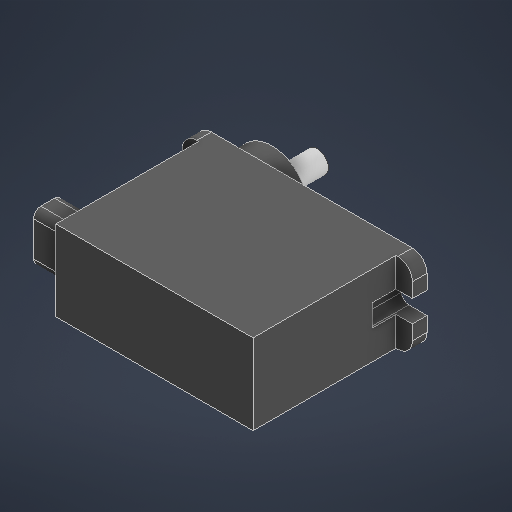
# Autodesk Inventor part: P_Servo_SIMPROP_27x12
Saved by Autodesk Inventor 2026 (Build 300175000, 175)
## iProperties
Created: 2025-08-29
Part Number: P_Servo_SIMPROP_27x12
Material: Generisch
Document SubType Name: Modeling
Designer: FAL
Density: 1 g/cm^3
Appearance: Vorgabe
Author: FAL
Autodesk Inventor part; units mm, degrees
ref_plane "YZ Plane" through (0, 0, 0) normal (1, 0, 0) x (0, 1, 0)
ref_plane "XZ Plane" through (0, 0, 0) normal (0, 1, 0) x (-1, 0, 0)
ref_plane "XY Plane" through (0, 0, 0) normal (0, 0, 1) x (1, 0, 0)
sketch "Skizze1" plane through (0, 0, 0) normal (0, 1, 0) x (-1, 0, 0)
  line L0 (-13.5, 5.5) -> (13.5, 5.5)
  line L1 (13.5, 5.5) -> (13.5, -5.5)
  line L2 (13.5, -5.5) -> (-13.5, -5.5)
  line L3 (-13.5, -5.5) -> (-13.5, 5.5)
  line L4 (-13.5, 5.5) -> (13.5, -5.5) construction
  line L5 (13.5, 5.5) -> (-13.5, -5.5) construction
  point P0 (0, 0)
  dimension "d0" = 27
  dimension "d1" = 11
  constraints: 12 end point, 2 midpoint, 2 parallel, 1 horizontal, 1 perpendicular
  measures "d0" distance of L0.start L0.end
  measures "d1" distance between parallel lines of L2 L0
extrude "Extrusion1" add sketch "Skizze1" along normal blind 21.55
sketch "Skizze2" plane through (0, 21.55, 0) normal (0, 1, 0) x (1, 0, 0)
  line L0 (15.75, -5.5) -> (-15.75, -5.5)
  line L1 (-15.75, -5.5) -> (-15.75, 5.5)
  line L2 (-15.75, 5.5) -> (15.75, 5.5)
  line L3 (15.75, 5.5) -> (15.75, -5.5)
  line L4 (15.75, -5.5) -> (-15.75, 5.5) construction
  line L5 (-15.75, -5.5) -> (15.75, 5.5) construction
  line L6 (13.5, 5.5) -> (-13.5, 5.5) projected
  point P0 (0, 0)
  dimension "d4" = 31.5
  constraints: 12 end point, 2 midpoint, 2 parallel, 1 collinear, 1 horizontal, 1 perpendicular
  measures "d4" distance between parallel lines of L3 L1
extrude "Extrusion2" add sketch "Skizze2" against normal blind 2
fillet "Rundung1" radius 2 4 edges at (-15.75, 20.55, 5.5) (15.75, 20.55, 5.5) (15.75, 20.55, -5.5) (-15.75, 20.55, -5.5)
sketch "Skizze3" plane through (0, 21.55, 0) normal (0, 1, 0) x (1, 0, 0)
  circle A0 centre (-8.5, 0) radius 5
  line L0 (-13.5, -5.5) -> (-13.5, 5.5) projected
  point P0 (0, 0)
  dimension "d8" = 5
  dimension "d9" = 10
  constraints: 1 centre point, 1 horizontal alignment
  measures "d8" distance from line of L0 A0.centre
  measures "d9" diameter of A0
extrude "Extrusion3" add sketch "Skizze3" along normal blind 3
sketch "Skizze4" plane through (-8.5, 24.55, 0) normal (0, 1, 0) x (1, 0, 0)
  circle A0 centre (0, 0) radius 1.5
  circle A1 centre (0, 0) radius 5 projected
  point P0 (8.5, 0)
  dimension "d12" = 3
  constraints: 1 centre point, 1 concentric
  measures "d12" diameter of A0
extrude "Extrusion4" add sketch "Skizze4" along normal blind 6.25 separate body contours A0
sketch "Skizze5" plane through (0, 21.55, 0) normal (0, 1, 0) x (1, 0, 0)
  line L0 (19.25, -1.5) -> (12.25, -1.5)
  line L1 (12.25, -1.5) -> (12.25, 1.5)
  line L2 (12.25, 1.5) -> (19.25, 1.5)
  line L3 (19.25, 1.5) -> (19.25, -1.5)
  line L4 (15.75, -3.5) -> (15.75, 3.5) projected
  line L5 (19.25, -1.5) -> (12.25, 1.5) construction
  line L6 (12.25, -1.5) -> (19.25, 1.5) construction
  line L7 (-12.25, -1.5) -> (-19.25, -1.5)
  line L8 (-19.25, -1.5) -> (-19.25, 1.5)
  line L9 (-19.25, 1.5) -> (-12.25, 1.5)
  line L10 (-12.25, 1.5) -> (-12.25, -1.5)
  line L11 (-15.75, -3.5) -> (-15.75, 3.5) projected
  line L12 (-12.25, -1.5) -> (-19.25, 1.5) construction
  line L13 (-19.25, -1.5) -> (-12.25, 1.5) construction
  point P0 (0, 0)
  point P1 (15.75, 0)
  point P2 (-15.75, 0)
  dimension "d15" = 3
  dimension "d16" = 3
  dimension "d17" = 3.5
  dimension "d18" = 3.5
  constraints: 24 end point, 6 midpoint, 4 parallel, 2 horizontal, 2 perpendicular
  measures "d15" distance between parallel lines of L2 L0
  measures "d16" distance between parallel lines of L9 L7
  measures "d17" distance between parallel lines of L11 L10
  measures "d18" distance between parallel lines of L4 L1
extrude "Extrusion5" cut sketch "Skizze5" against normal blind 5.25 bodies 1
fillet "Rundung2" radius 1 4 edges at (-12.25, 18.925, 1.5) (-12.25, 18.925, -1.5) (12.25, 18.925, 1.5) (12.25, 18.925, -1.5)
sketch "Skizze6" plane through (-13.5, 0, -5.5) normal (-1, 0, 0) x (0, 0, 1)
  line L0 (2.1189, 6.0927) -> (8.8811, 6.0927)
  line L1 (8.8811, 6.0927) -> (8.8811, 2.2095)
  line L2 (8.8811, 2.2095) -> (2.1189, 2.2095)
  line L3 (2.1189, 2.2095) -> (2.1189, 6.0927)
  line L4 (2.1189, 6.0927) -> (8.8811, 2.2095) construction
  line L5 (8.8811, 6.0927) -> (2.1189, 2.2095) construction
  point P0 (5.5, 0)
  point P1 (5.5, 4.1511)
  constraints: 12 end point, 2 midpoint, 2 parallel, 1 horizontal, 1 perpendicular
extrude "Extrusion6" add sketch "Skizze6" along normal blind 5.25 bodies 1
fillet "Rundung3" radius 1 4 edges at (-16.125, 6.0927, -3.3811) (-16.125, 2.2095, -3.3811) (-16.125, 2.2095, 3.3811) (-16.125, 6.0927, 3.3811)
fillet "Rundung4" radius 1 8 edges at (-13.5, 5.7998, 3.0882) (-13.5, 4.1511, 3.3811) (-13.5, 2.5023, 3.0882) (-13.5, 2.2095, 0) (-13.5, 2.5023, -3.0882) (-13.5, 4.1511, -3.3811) (-13.5, 5.7998, -3.0882) (-13.5, 6.0927, 0)
